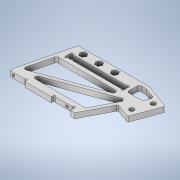
# Autodesk Inventor part: Trunk_lower_flank_frame
Saved by Autodesk Inventor 2020.4 (Build 244396000, 396)
## iProperties
Created: 2021-09-11
Part Number: Trunk_lower_flank_frame
Material: アルミニウム 2014-T4
Document SubType Name: Modeling
Designer: Masato Kubotera
Density: 2.8 g/cm^3
Appearance: 滑らか - 淡い灰色
Mass: 32.437 g
Surface Area: 89.3164 cm^2
Volume: 11.5847 cm^3
Description: A2017 T5
Author: Masato Kubotera
Autodesk Inventor part; units mm, degrees
ref_plane "YZ Plane" through (0, 0, 0) normal (1, 0, 0) x (0, 1, 0)
ref_plane "XZ Plane" through (0, 0, 0) normal (0, 1, 0) x (-1, 0, 0)
ref_plane "XY Plane" through (0, 0, 0) normal (0, 0, 1) x (1, 0, 0)
derived "Trunk_vertical_frame_03.ipt"
sketch "スケッチ1" plane through (0, 0, 0) normal (0, 0, 1) x (1, 0, 0)
  circle A0 centre (0, 0) radius 11
  line L0 (1, 13.5) -> (28, 13.5) construction
  line L1 (28, 13.5) -> (28, -13.5) construction
  line L2 (28, -13.5) -> (1, -13.5) construction
  line L3 (1, -13.5) -> (1, 13.5) construction
  line L4 (1, 13.5) -> (28, -13.5) construction
  line L5 (28, 13.5) -> (1, -13.5) construction
  line L6 (-12, 16) -> (39.5, 16) construction
  line L7 (39.5, 16) -> (39.5, -16) construction
  line L8 (39.5, -16) -> (-12, -16) construction
  line L9 (-12, -16) -> (-12, 16) construction
  line L10 (-12, 16) -> (39.5, -16) construction
  line L11 (39.5, 16) -> (-12, -16) construction
  circle A1 centre (1, 13.5) radius 1.35
  arc A2 (0, 16) -> (-12, 10.583) centre (0, 0) ccw construction
  line L12 (-12, 0) -> (39.5, 0)
  circle A3 centre (28, 13.5) radius 1.35
  arc A4 (-12, -10.583) -> (0, -16) centre (0, 0) ccw construction
  circle A5 centre (28, -13.5) radius 1.35
  circle A6 centre (1, -13.5) radius 1.35
  arc A7 (0, 16.01) -> (-12.01, 10.5868) centre (0, 0) ccw
  line L13 (0, 16.01) -> (39.51, 16.01)
  line L14 (39.51, 16.01) -> (39.51, 13.26)
  line L15 (-12.01, 10.5868) -> (-12.01, 0)
  arc A8 (-11.4729, 11.1666) -> (-12.01, 9.8444) centre (-11.0278, 10.2156) ccw
  line L16 (-12.01, 10.5868) -> (-11.0278, 10.2156) construction
  arc A9 (39.51, 14.5251) -> (38.0251, 16.01) centre (38.7675, 15.2675) ccw
  line L17 (38.7675, 15.2675) -> (39.51, 16.01) construction
  arc A10 (38.0251, -16.01) -> (39.51, -14.5251) centre (38.7675, -15.2675) ccw
  line L18 (-12.01, -10.5868) -> (-12.01, 0)
  arc A11 (-12.01, -9.8444) -> (-11.4729, -11.1666) centre (-11.0278, -10.2156) ccw
  arc A12 (-12.01, -10.5868) -> (0, -16.01) centre (0, 0) ccw
  line L19 (0, -16.01) -> (39.51, -16.01)
  line L20 (39.51, 13.26) -> (42.01, 13.26)
  line L21 (42.01, 13.26) -> (42.01, -1.76)
  line L22 (42.01, -1.76) -> (39.51, -1.76)
  line L23 (39.51, -1.76) -> (39.51, -14.5251)
  line L24 (39.5, 13.25) -> (42, 13.25) construction
  line L25 (42, 13.25) -> (42, -1.75) construction
  line L26 (42, -1.75) -> (39.5, -1.75) construction
  line L27 (42, 5.75) -> (39.5, 5.75) construction
  arc A13 (42.01, 11.7751) -> (40.5251, 13.26) centre (41.2675, 12.5175) ccw
  line L28 (41.2675, 12.5175) -> (42.01, 13.26) construction
  arc A14 (40.5251, -1.76) -> (42.01, -0.2751) centre (41.2675, -1.0175) ccw
  circle A15 centre (-15.5, 19) radius 1.55
  line L29 (-18, 22) -> (-13, 22) construction
  line L30 (-13, 22) -> (-13, -10.5) construction
  line L31 (-13, -10.5) -> (-18, -10.5) construction
  line L32 (-18, -10.5) -> (-18, 22) construction
  line L33 (-18, 22) -> (-13, -10.5) construction
  line L34 (-13, 22) -> (-18, -10.5) construction
  line L35 (-18, 5.75) -> (-13, 5.75) construction
  line L36 (-15.5, 22) -> (-15.5, -10.5) construction
  line L37 (-18, 13.25) -> (-15.5, 13.25) construction
  line L38 (-15.5, 13.25) -> (-15.5, -1.75) construction
  line L39 (-15.5, -1.75) -> (-18, -1.75) construction
  line L40 (-18, 13.25) -> (-15.5, -1.75) construction
  line L41 (-15.5, 13.25) -> (-18, -1.75) construction
  line L42 (-15.49, -1.76) -> (-18.01, -1.76)
  line L43 (-18.01, -1.76) -> (-18.01, 13.26)
  line L44 (-18.01, 13.26) -> (-15.49, 13.26)
  line L45 (-15.49, 13.26) -> (-15.49, -1.76)
  line L46 (-15.49, -1.76) -> (-18.01, 13.26) construction
  line L47 (-18.01, -1.76) -> (-15.49, 13.26) construction
  line L48 (-16.75, 13.26) -> (-16.75, -1.76) construction
  arc A16 (-18.01, 13.26) -> (-18.01, 11.16) centre (-18.01, 12.21) ccw
  arc A17 (-15.49, 11.16) -> (-15.49, 13.26) centre (-15.49, 12.21) ccw
  arc A18 (-18.01, 0.34) -> (-18.01, -1.76) centre (-18.01, -0.71) ccw
  arc A19 (-15.49, -1.76) -> (-15.49, 0.34) centre (-15.49, -0.71) ccw
  circle A20 centre (-15.5, -7.5) radius 1.55
  line L49 (14.5, 16) -> (14.5, -16) construction
  circle A21 centre (42, 19) radius 1.55
  line L50 (39.5, 22) -> (44.5, 22) construction
  line L51 (44.5, 22) -> (44.5, -10.5) construction
  line L52 (44.5, -10.5) -> (39.5, -10.5) construction
  line L53 (39.5, 22) -> (44.5, -10.5) construction
  line L54 (44.5, 22) -> (39.5, -10.5) construction
  line L55 (42, 22) -> (42, -10.5) construction
  circle A22 centre (42, -7.5) radius 1.55
  line L56 (-12, -18.25) -> (27, -18.25) construction
  line L57 (27, -18.25) -> (27, -23.25) construction
  line L58 (27, -23.25) -> (-12, -23.25) construction
  line L59 (-12, -23.25) -> (-12, -18.25) construction
  line L60 (-12, -18.25) -> (27, -23.25) construction
  line L61 (27, -18.25) -> (-12, -23.25) construction
  line L62 (-3, -20.75) -> (18, -20.75) construction
  line L63 (18, -20.75) -> (18, -18.25) construction
  line L64 (-3, -18.25) -> (-3, -20.75) construction
  line L65 (-3, -20.75) -> (18, -18.25) construction
  line L66 (18, -20.75) -> (-3, -18.25) construction
  line L67 (-12, -20.75) -> (27, -20.75) construction
  line L68 (7.5, -18.25) -> (7.5, -23.25) construction
  line L69 (-3.01, -18.24) -> (18.01, -18.24)
  line L70 (18.01, -18.24) -> (18.01, -20.76)
  line L71 (18.01, -20.76) -> (-3.01, -20.76)
  line L72 (-3.01, -20.76) -> (-3.01, -18.24)
  line L73 (-3.01, -18.24) -> (18.01, -20.76) construction
  line L74 (18.01, -18.24) -> (-3.01, -20.76) construction
  circle A23 centre (-8, -20.75) radius 1.55
  circle A24 centre (23, -20.75) radius 1.55
  arc A25 (-0.91, -18.24) -> (-3.01, -18.24) centre (-1.96, -18.24) ccw
  arc A26 (18.01, -18.24) -> (15.91, -18.24) centre (16.96, -18.24) ccw
  line L75 (-3.01, -19.5) -> (18.01, -19.5) construction
  arc A27 (-3.01, -20.76) -> (-0.91, -20.76) centre (-1.96, -20.76) ccw
  arc A28 (15.91, -20.76) -> (18.01, -20.76) centre (16.96, -20.76) ccw
  circle A29 centre (-8, 20.75) radius 1.55
  line L76 (18.01, 20.76) -> (-3.01, 20.76)
  line L77 (-3.01, 19.5) -> (18.01, 19.5) construction
  line L78 (-3, 18.25) -> (-3, 20.75) construction
  line L79 (18, 20.75) -> (-3, 18.25) construction
  line L80 (-3, 20.75) -> (18, 18.25) construction
  line L81 (-3.01, 20.76) -> (-3.01, 18.24)
  line L82 (-3.01, 18.24) -> (18.01, 20.76) construction
  line L83 (-3.01, 18.24) -> (18.01, 18.24)
  arc A30 (-3.01, 18.24) -> (-0.91, 18.24) centre (-1.96, 18.24) ccw
  line L84 (18.01, 18.24) -> (-3.01, 20.76) construction
  line L85 (-12, 23.25) -> (-12, 18.25) construction
  arc A31 (-0.91, 20.76) -> (-3.01, 20.76) centre (-1.96, 20.76) ccw
  line L86 (7.5, 18.25) -> (7.5, 23.25) construction
  line L87 (-3, 20.75) -> (18, 20.75) construction
  line L88 (-12, 20.75) -> (27, 20.75) construction
  line L89 (27, 23.25) -> (-12, 23.25) construction
  line L90 (-12, 18.25) -> (27, 18.25) construction
  line L91 (-12, 18.25) -> (27, 23.25) construction
  line L92 (27, 18.25) -> (-12, 23.25) construction
  line L93 (27, 18.25) -> (27, 23.25) construction
  arc A32 (15.91, 18.24) -> (18.01, 18.24) centre (16.96, 18.24) ccw
  circle A33 centre (23, 20.75) radius 1.55
  line L94 (18, 20.75) -> (18, 18.25) construction
  line L95 (18.01, 18.24) -> (18.01, 20.76)
  arc A34 (18.01, 20.76) -> (15.91, 20.76) centre (16.96, 20.76) ccw
  line L96 (-18, 28.25) -> (44.5, 28.25)
  line L97 (-18, 28.25) -> (-23, 22)
  line L98 (44.5, 28.25) -> (47.5, 22)
  line L99 (-23, 22) -> (-23, -2.875)
  line L100 (47.5, 22) -> (47.5, -18.25)
  line L101 (47.5, -18.25) -> (37, -33.25)
  line L102 (-23, -2.875) -> (-33.5, -16)
  line L103 (-33.5, -16) -> (-33.5, -87)
  line L104 (37, -33.25) -> (37, -70.3333)
  line L105 (37, -70.3333) -> (23, -96) construction
  line L106 (23, -96) -> (-17, -96) construction
  line L107 (-17, -96) -> (-33.5, -87) construction
  circle A35 centre (-12, -91) radius 1.55
  circle A36 centre (3, -91) radius 1.55
  line L108 (-17, -96) -> (-17, -86) construction
  line L109 (-17, -86) -> (23, -86) construction
  line L110 (23, -86) -> (23, -96) construction
  line L111 (-17, -91) -> (23, -91) construction
  line L112 (3, -86) -> (3, -96) construction
  circle A37 centre (18, -91) radius 1.55
  circle A38 centre (-13.5, -53.25) radius 1.55
  line L113 (-23.5, -57.25) -> (27, -57.25)
  line L114 (27, -57.25) -> (27, -76)
  line L115 (27, -76) -> (-23.5, -76)
  line L116 (-23.5, -76) -> (-23.5, -57.25)
  line L117 (-23.5, -33.25) -> (27, -33.25)
  line L118 (27, -33.25) -> (27, -49.25)
  line L119 (27, -49.25) -> (-23.5, -49.25)
  line L120 (-23.5, -49.25) -> (-23.5, -33.25)
  circle A39 centre (-13.5, -53.25) radius 4 construction
  arc A40 (-11.4565, -93.76) -> (-9.8815, -92.8507) centre (-10.9315, -92.8507) ccw
  line L121 (-9.338, -91.9093) -> (-9.8815, -92.8507)
  arc A41 (-9.338, -91.9093) -> (-9.338, -90.0907) centre (-9.863, -91) ccw
  line L122 (-9.8815, -89.1493) -> (-9.338, -90.0907)
  arc A42 (-9.8815, -89.1493) -> (-11.4565, -88.24) centre (-10.9315, -89.1493) ccw
  line L123 (-12.5435, -88.24) -> (-11.4565, -88.24)
  arc A43 (-12.5435, -88.24) -> (-14.1185, -89.1493) centre (-13.0685, -89.1493) ccw
  line L124 (-14.662, -90.0907) -> (-14.1185, -89.1493)
  arc A44 (-14.662, -90.0907) -> (-14.662, -91.9093) centre (-14.137, -91) ccw
  line L125 (-14.1185, -92.8507) -> (-14.662, -91.9093)
  arc A45 (-14.1185, -92.8507) -> (-12.5435, -93.76) centre (-13.0685, -92.8507) ccw
  line L126 (-11.4565, -93.76) -> (-12.5435, -93.76)
  arc A46 (5.662, -91.9093) -> (5.662, -90.0907) centre (5.137, -91) ccw
  line L127 (5.1185, -89.1493) -> (5.662, -90.0907)
  line L128 (5.662, -91.9093) -> (5.1185, -92.8507)
  arc A47 (3.5435, -93.76) -> (5.1185, -92.8507) centre (4.0685, -92.8507) ccw
  arc A48 (5.1185, -89.1493) -> (3.5435, -88.24) centre (4.0685, -89.1493) ccw
  line L129 (2.4565, -88.24) -> (3.5435, -88.24)
  arc A49 (2.4565, -88.24) -> (0.8815, -89.1493) centre (1.9315, -89.1493) ccw
  line L130 (0.338, -90.0907) -> (0.8815, -89.1493)
  arc A50 (0.338, -90.0907) -> (0.338, -91.9093) centre (0.863, -91) ccw
  line L131 (0.8815, -92.8507) -> (0.338, -91.9093)
  arc A51 (0.8815, -92.8507) -> (2.4565, -93.76) centre (1.9315, -92.8507) ccw
  line L132 (3.5435, -93.76) -> (2.4565, -93.76)
  arc A52 (20.662, -91.9093) -> (20.662, -90.0907) centre (20.137, -91) ccw
  line L133 (20.1185, -89.1493) -> (20.662, -90.0907)
  line L134 (20.662, -91.9093) -> (20.1185, -92.8507)
  arc A53 (18.5435, -93.76) -> (20.1185, -92.8507) centre (19.0685, -92.8507) ccw
  arc A54 (20.1185, -89.1493) -> (18.5435, -88.24) centre (19.0685, -89.1493) ccw
  line L135 (17.4565, -88.24) -> (18.5435, -88.24)
  arc A55 (17.4565, -88.24) -> (15.8815, -89.1493) centre (16.9315, -89.1493) ccw
  line L136 (15.338, -90.0907) -> (15.8815, -89.1493)
  arc A56 (15.338, -90.0907) -> (15.338, -91.9093) centre (15.863, -91) ccw
  line L137 (15.8815, -92.8507) -> (15.338, -91.9093)
  arc A57 (15.8815, -92.8507) -> (17.4565, -93.76) centre (16.9315, -92.8507) ccw
  line L138 (18.5435, -93.76) -> (17.4565, -93.76)
  line L139 (-33.5, -86) -> (46, -86)
  line L140 (46, -86) -> (46, -115.797) construction
  line L141 (46, -115.797) -> (32.99, -141)
  line L142 (-33.5, -86) -> (-33.5, -139)
  line L143 (-33.5, -139) -> (28, -139)
  arc A58 (-17.5, -139) -> (-19.6, -139) centre (-18.55, -139) ccw
  line L144 (-17.5, -139) -> (-17.5, -141)
  line L145 (7.5, -141) -> (7.5, -139)
  arc A59 (9.6, -139) -> (7.5, -139) centre (8.55, -139) ccw
  line L146 (-30.5, -139) -> (-30.5, -141) construction
  line L147 (-33.5, -139) -> (-33.5, -141) construction
  line L148 (27.99, -139) -> (27.99, -141) construction
  line L149 (24.99, -139) -> (24.99, -141) construction
  line L150 (-33.5, -141) -> (7.5, -141) construction
  line L151 (7.5, -141) -> (32.99, -141) construction
  line L152 (28, -139) -> (34.0224, -139) construction
  arc A60 (28, -139) -> (25.9, -139) centre (26.95, -139) ccw
  line L153 (-19, -96) -> (36.5, -96) construction
  line L154 (36.5, -96) -> (36.5, -101) construction
  line L155 (36.5, -101) -> (-19, -101) construction
  line L156 (-19, -101) -> (-19, -96) construction
  line L157 (-19, -98.5) -> (36.5, -98.5) construction
  line L158 (8.75, -96) -> (8.75, -101) construction
  line L159 (-19.05, -95.95) -> (36.55, -95.95)
  line L160 (36.55, -95.95) -> (36.55, -101.05)
  line L161 (36.55, -101.05) -> (-19.05, -101.05)
  line L162 (-19.05, -101.05) -> (-19.05, -95.95)
  line L163 (-19.05, -95.95) -> (36.55, -101.05) construction
  line L164 (36.55, -95.95) -> (-19.05, -101.05) construction
  arc A61 (-16.95, -95.95) -> (-19.05, -95.95) centre (-18, -95.95) ccw
  arc A62 (36.55, -95.95) -> (34.45, -95.95) centre (35.5, -95.95) ccw
  arc A63 (-19.05, -101.05) -> (-16.95, -101.05) centre (-18, -101.05) ccw
  arc A64 (34.45, -101.05) -> (36.55, -101.05) centre (35.5, -101.05) ccw
  line L165 (46, -86) -> (69.5821, -94.5832)
  line L166 (69.5821, -94.5832) -> (60.0056, -120.8946)
  line L167 (60.0056, -120.8946) -> (46, -115.797)
  line L168 (46, -100.8985) -> (64.7939, -107.7389) construction
  circle A65 centre (61.8919, -98.1692) radius 6 construction
  line L169 (61.8919, -98.1692) -> (59.1557, -105.6868) construction
  circle A66 centre (61.8919, -98.1692) radius 2.25
  line L170 (60.8018, -101.164) -> (58.7533, -98.7226) construction
  line L171 (58.7533, -98.7226) -> (59.8433, -95.7279) construction
  line L172 (59.8433, -95.7279) -> (62.9819, -95.1745) construction
  line L173 (62.9819, -95.1745) -> (65.0304, -97.6158) construction
  line L174 (65.0304, -97.6158) -> (63.9404, -100.6106) construction
  line L175 (63.9404, -100.6106) -> (60.8018, -101.164) construction
  arc A67 (60.1269, -100.3597) -> (61.8359, -100.9817) centre (61.161, -100.1773) ccw
  arc A68 (62.9064, -100.7929) -> (64.2995, -99.6239) centre (63.2655, -99.8062) ccw construction
  arc A69 (64.6713, -98.6025) -> (64.3555, -96.8115) centre (63.9964, -97.7981) ccw construction
  arc A70 (63.6568, -95.9788) -> (61.9478, -95.3568) centre (62.6227, -96.1611) ccw construction
  arc A71 (60.8774, -95.5455) -> (59.4842, -96.7145) centre (60.5182, -96.5322) ccw construction
  arc A72 (59.1124, -97.736) -> (59.4282, -99.527) centre (59.7873, -98.5403) ccw construction
  circle A73 centre (56.4195, -113.2043) radius 2.25
  line L176 (57.5095, -110.2095) -> (54.371, -110.7629) construction
  line L177 (54.371, -110.7629) -> (53.281, -113.7577) construction
  line L178 (53.281, -113.7577) -> (55.3295, -116.1991) construction
  line L179 (55.3295, -116.1991) -> (58.4681, -115.6457) construction
  line L180 (58.4681, -115.6457) -> (59.5581, -112.6509) construction
  line L181 (59.5581, -112.6509) -> (57.5095, -110.2095) construction
  arc A74 (58.1845, -111.0139) -> (56.4755, -110.3919) centre (57.1504, -111.1962) ccw construction
  arc A75 (59.199, -113.6376) -> (58.8832, -111.8466) centre (58.524, -112.8332) ccw construction
  arc A76 (57.434, -115.828) -> (58.8272, -114.659) centre (57.7932, -114.8413) ccw construction
  arc A77 (54.6546, -115.3947) -> (56.3636, -116.0168) centre (55.6886, -115.2124) ccw construction
  arc A78 (53.6401, -112.771) -> (53.9559, -114.5621) centre (54.315, -113.5754) ccw construction
  arc A79 (55.405, -110.5806) -> (54.0119, -111.7496) centre (55.0459, -111.5673) ccw construction
  line L182 (47.1779, -106.9749) -> (33.2273, -134)
  line L183 (33.2273, -134) -> (-26.0778, -134)
  line L184 (-26.0778, -134) -> (47.1779, -106.9749)
  line L185 (-29.982, -132.2427) -> (43.8635, -105)
  line L186 (43.8635, -105) -> (-23.3215, -105)
  line L187 (-23.3215, -105) -> (-29.982, -132.2427)
  line L188 (-21.7646, -86) -> (-33.5, -134)
  line L189 (-30.4116, -134) -> (48.1974, -105) construction
  line L190 (-26.0778, -134) -> (-33.5, -134) construction
  line L191 (28, -143) -> (31.9576, -143)
  line L192 (28, -139) -> (28, -143)
  line L193 (32.99, -141) -> (31.9576, -143)
  circle A80 centre (56.4195, -113.2043) radius 6 construction
  line L194 (39.5, -101) -> (39.5, -89.1925)
  line L195 (39.5, -89.1925) -> (46, -89.1925)
  line L196 (46, -89.1925) -> (57.2798, -93.298)
  line L197 (57.2798, -93.298) -> (54.4765, -101)
  line L198 (54.4765, -101) -> (39.5, -101)
  circle A81 centre (61.8919, -98.1692) radius 1.55 construction
  circle A82 centre (56.4195, -113.2043) radius 1.55 construction
  line L199 (-17.5, -141) -> (7.5, -141)
  point P0 (14.5, 0)
  point P1 (-15.5, 5.75)
  point P2 (-16.75, 5.75)
  point P3 (14.5, 0)
  point P4 (42, 5.75)
  point P5 (42, 5.75)
  point P6 (7.5, -20.75)
  point P7 (7.5, -19.5)
  point P8 (7.5, -19.5)
  point P9 (7.5, -19.5)
  point P10 (7.5, -19.5)
  point P11 (7.5, 20.75)
  point P12 (7.5, 19.5)
  point P13 (7.5, 19.5)
  point P14 (7.5, 19.5)
  point P15 (7.5, 19.5)
  point P16 (-10.4065, -93.76)
  point P17 (-8.813, -91)
  point P18 (-10.4065, -88.24)
  point P19 (-13.5935, -88.24)
  point P20 (-13.5935, -88.24)
  point P21 (-15.187, -91)
  point P22 (-13.5935, -93.76)
  point P23 (-15.187, -91)
  point P24 (-8.813, -91)
  point P25 (3, -91)
  point P26 (6.187, -91)
  point P27 (6.187, -91)
  point P28 (4.5935, -88.24)
  point P29 (4.5935, -93.76)
  point P30 (3, -91)
  point P31 (3, -91)
  point P32 (1.4065, -88.24)
  point P33 (1.4065, -88.24)
  point P34 (-0.187, -91)
  point P35 (-0.187, -91)
  point P36 (1.4065, -93.76)
  point P37 (18, -91)
  point P38 (21.187, -91)
  point P39 (21.187, -91)
  point P40 (19.5935, -88.24)
  point P41 (19.5935, -93.76)
  point P42 (18, -91)
  point P43 (18, -91)
  point P44 (16.4065, -88.24)
  point P45 (16.4065, -88.24)
  point P46 (14.813, -91)
  point P47 (14.813, -91)
  point P48 (16.4065, -93.76)
  point P49 (3, -86)
  point P50 (8.75, -98.5)
  point P51 (63.9404, -100.6106)
  point P52 (65.0304, -97.6158)
  point P53 (62.9819, -95.1745)
  point P54 (59.8433, -95.7279)
  point P55 (58.7533, -98.7226)
  point P56 (59.5581, -112.6509)
  point P57 (58.4681, -115.6457)
  point P58 (55.3295, -116.1991)
  point P59 (53.281, -113.7577)
  point P60 (54.371, -110.7629)
  point P61 (34.45, -101.05)
  point P62 (-16.95, -101.05)
  point P63 (34.45, -95.95)
  point P64 (-14.1185, -89.1493)
  point P65 (0.8815, -89.1493)
  point P66 (15.8815, -89.1493)
  point P67 (57.434, -115.828)
  point P68 (56.3636, -116.0168)
  point P69 (54.6546, -115.3947)
  point P70 (53.9559, -114.5621)
  point P71 (53.6401, -112.771)
  point P72 (54.0119, -111.7496)
  point P73 (55.405, -110.5806)
  point P74 (58.8832, -111.8466)
  point P75 (59.199, -113.6376)
  point P76 (58.8272, -114.659)
  point P77 (59.1124, -97.736)
  point P78 (59.4842, -96.7145)
  point P79 (60.8774, -95.5455)
  point P80 (61.9478, -95.3568)
  point P81 (63.6568, -95.9788)
  point P82 (64.3555, -96.8115)
  point P83 (64.6713, -98.6025)
  point P84 (64.2995, -99.6239)
  point P85 (62.9064, -100.7929)
  point P86 (59.4282, -99.527)
  point P87 (7.5, -139)
  point P88 (7.5, -139)
  dimension "d2" = 1.05
  dimension "d7" = 1.05
  dimension "d12" = 2
  dimension "d16" = 3
  dimension "d17" = 3
  dimension "d22" = 5
  dimension "d23" = 1.05
  dimension "d24" = 43
  dimension "d25" = 43
  dimension "d27" = 0.05
  dimension "d28" = 0.05
  dimension "d29" = 5
  dimension "d30" = 55.5
  dimension "d31" = 1.05
  dimension "d33" = 22
  dimension "d34" = 12
  dimension "d36" = 4.5
  dimension "d37" = 5.52
  dimension "d38" = 1.05
  dimension "d41" = 360
  dimension "d43" = 16
  dimension "d44" = 3
  dimension "d47" = 5
  dimension "d48" = 4
  dimension "d50" = 3
  dimension "d52" = 1.5
  dimension "d53" = 1.5
  dimension "d55" = 5
  dimension "d73" = 5
  dimension "d74" = 4
  dimension "d75" = 0.01
  dimension "d76" = 110
  dimension "d77" = 20
  dimension "d78" = 3
  dimension "d79" = 3
  dimension "d80" = 3.1
  dimension "d83" = 25
  dimension "d84" = 16
  dimension "d88" = 61.5
  measures "d2" radius of A58
  measures "d7" radius of A59
  measures "d12" distance of L142.end L147.end
  measures "d16" distance of L147.end L146.end
  measures "d17" distance of L148.end L149.end
  measures "d22" distance of L141.end L148.end
  measures "d23" radius of A60
  measures "d24" vertical distance of L142.end L106.end
  measures "d25" distance of L139.end L112.start
  measures "d27" horizontal distance of L159.start L153.start
  measures "d28" horizontal distance of L153.start L159.start
  measures "d29" distance of L155.end L153.start
  measures "d30" distance of L157.end L157.start
  measures "d31" radius of A61
  measures "d33" horizontal distance of L153.start point (3, -91)
  measures "d34" diameter of A65
  measures "d36" diameter of A66
  measures "d37" distance from line of L172 L174.end
  measures "d38" radius of A67
  measures "d43" distance of point (56.42, -113.204) A66.centre
  measures "d44" distance between parallel lines of L141 L182
  measures "d47" distance of L188.end L142.end
  measures "d48" vertical distance of L186.end L155.end
  measures "d50" distance between parallel lines of L188 L187
  measures "d52" distance between parallel lines of L184 L189
  measures "d53" distance between parallel lines of L189 L185
  measures "d55" distance from line of L159.start L188
  measures "d73" vertical distance of A35.centre L153.start
  measures "d74" distance between parallel lines of L191 L152
  measures "d75" distance between parallel lines of L192 L148
  measures "d76" angle of L140 L168
  measures "d77" distance of L168.start L168.end
  measures "d78" distance between parallel lines of L196 L165
  measures "d79" distance between parallel lines of L154 L194
  measures "d80" diameter of A81
  measures "d83" distance of L145.start L144.end
  measures "d84" horizontal distance of L144.end L142.end
  measures "d88" horizontal distance of L142.end L191.start
extrude "押し出し1" add sketch "スケッチ1" along normal blind 5 contours L139 L165 L166 L167 L141 L193 L191 L192 A60 L143 A59 A58 L142 L188 | L143 L145 L199 L144
sketch "スケッチ2" plane through (-33.5, -139, 0) normal (0, -1, 0) x (1, 0, 0)
  line L0 (41, 0) -> (41, 5) projected
  line L1 (61.5, 0) -> (61.5, 5) projected
  line L2 (16, 0) -> (16, 5) projected
  point P0 (33.5, 0)
  point P1 (3, 2.5)
  point P2 (0, 0)
  point P3 (54, 2.5)
  dimension "d59" = 2.5
  dimension "d61" = 2.5
  dimension "d86" = 13
  dimension "d87" = 13
  measures "d59" vertical distance of point (0, 0) point (3, 2.5)
  measures "d61" vertical distance of point (0, 0) point (54, 2.5)
  measures "d86" distance from line of point (3, 2.5) L2
  measures "d87" distance from line of point (54, 2.5) L0
hole "穴1" at (-30.5, -139, 2.5) at (20.5, -139, 2.5) direction (0, 1, 0) diameter 2.459 depth 5 thread size "M3x0.5" class "6H" standard "ISO Metric profile"
fillet "フィレット1" radius 1 6 edges at (-21.7646, -86, 2.5) (69.5821, -94.5832, 2.5) (60.0056, -120.8946, 2.5) (46, -115.797, 2.5) (46, -86, 2.5) (-33.5, -134, 2.5)
fillet "フィレット2" radius 2 10 edges at (-23.3215, -105, 2.5) (-29.982, -132.2427, 2.5) (-26.0778, -134, 2.5) (43.8635, -105, 2.5) (33.2273, -134, 2.5) (47.1779, -106.9749, 2.5) (39.5, -89.1925, 2.5) (39.5, -101, 2.5) (54.4765, -101, 2.5) (57.2798, -93.298, 2.5)
equation "\"d7\" = d2"
equation "\"d23\" = d7"
equation "\"d28\" = d27"
equation "\"d31\" = d2"
equation "\"d38\" = d2"
equation "\"d50\" = d49"
equation "\"d13\" = d10"
equation "\"d49\" = 3"
equation "\"d10\" = 0.01"
